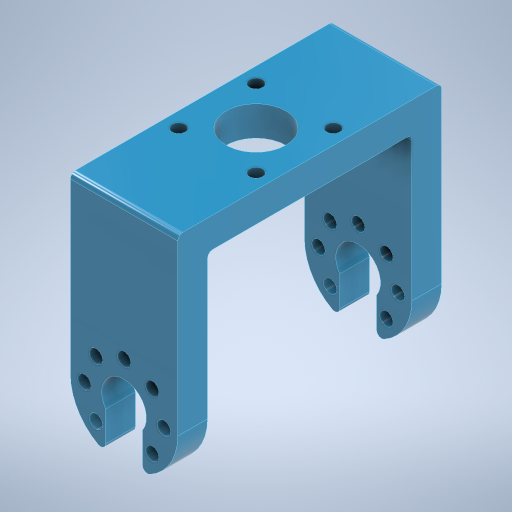
# Autodesk Inventor part: 3D_upper_to_arm1
Saved by Autodesk Inventor 2024 (Build 280153000, 153)
## iProperties
Created: 2024-09-07
Part Number: 3D_upper_to_arm1
Material: PMMA 플라스틱
Document SubType Name: Modeling
Designer: jmha0
Density: 1.188 g/cm^3
Appearance: 하늘색 짙음
Author: jmha0
Autodesk Inventor part; units mm, degrees
ref_plane "YZ Plane" through (0, 0, 0) normal (1, 0, 0) x (0, 1, 0)
ref_plane "XZ Plane" through (0, 0, 0) normal (0, 1, 0) x (-1, 0, 0)
ref_plane "XY Plane" through (0, 0, 0) normal (0, 0, 1) x (1, 0, 0)
sketch "스케치1" plane through (0, 0, 0) normal (0, 0, 1) x (1, 0, 0)
  circle A0 centre (-22.9272, 17.0843) radius 10.8
  circle A1 centre (-22.9272, 17.0843) radius 6
  circle A2 centre (-22.9272, 9.0843) radius 1.05
  circle A3 centre (-28.584, 11.4274) radius 1.05
  circle A4 centre (-30.9272, 17.0843) radius 1.05
  circle A5 centre (-28.584, 22.7411) radius 1.05
  circle A6 centre (-22.9272, 25.0843) radius 1.05
  circle A7 centre (-17.2703, 22.7411) radius 1.05
  circle A8 centre (-14.9272, 17.0843) radius 1.05
  circle A9 centre (-17.2703, 11.4274) radius 1.05
  circle A10 centre (-28.584, 22.7411) radius 1.15
  circle A11 centre (-22.9272, 25.0843) radius 1.15
  circle A12 centre (-17.2703, 22.7411) radius 1.15
  circle A13 centre (-14.9272, 17.0843) radius 1.15
  circle A14 centre (-17.2703, 11.4274) radius 1.15
  circle A15 centre (-28.584, 11.4274) radius 1.15
  circle A16 centre (-30.9272, 17.0843) radius 1.15
  circle A17 centre (-22.9272, 17.0843) radius 3.5
  arc A18 (-19.2272, 17.0843) -> (-26.6272, 17.0843) centre (-22.9272, 17.0843) ccw
  arc A19 (-19.2272, 6.9378) -> (-26.6272, 6.9378) centre (-22.9272, 17.0843) ccw
  line L0 (-26.6272, 17.0843) -> (-26.6272, 6.9378)
  line L1 (-19.2272, 17.0843) -> (-19.2272, 6.9378)
  line L2 (-33.7272, 17.0843) -> (-33.7272, 52.0843)
  line L3 (-12.1272, 17.0843) -> (-12.1272, 52.0843)
  line L4 (-12.1272, 52.0843) -> (-33.7272, 52.0843)
  line L5 (-33.7272, 52.0843) -> (-12.1272, 52.0843)
  line L6 (-12.1272, 52.0843) -> (-12.1272, 58.0843)
  line L7 (-12.1272, 58.0843) -> (-33.7272, 58.0843)
  line L8 (-33.7272, 58.0843) -> (-33.7272, 52.0843)
  point P0 (0, 0)
  dimension "d0" = 0.1
  dimension "d1" = 0.1
  dimension "d2" = 0.1
  dimension "d3" = 0.1
  dimension "d4" = 0.1
  dimension "d5" = 0.1
  dimension "d6" = 0.1
  dimension "d7" = 0.2
  dimension "d8" = 35
  dimension "d9" = 35
  dimension "d10" = 6
  constraints: 20 centre point, 18 end point, 6 point on circle, 6 tangent, 4 parallel, 2 vertical, 1 coincident, 1 concentric, 1 horizontal, 1 perpendicular
  measures "d0" radial gap between concentric circles of A5 A10
  measures "d1" radial gap between concentric circles of A6 A11
  measures "d2" radial gap between concentric circles of A7 A12
  measures "d3" radial gap between concentric circles of A8 A13
  measures "d4" radial gap between concentric circles of A9 A14
  measures "d5" radial gap between concentric circles of A3 A15
  measures "d6" radial gap between concentric circles of A4 A16
  measures "d7" radial gap between concentric circles of A17 A18
  measures "d8" distance of L2.start L4.end
  measures "d9" distance of L3.start L3.end
  measures "d10" distance of L6.end L5.end
extrude "돌출1" add sketch "스케치1" along normal blind 6 contours A0 L1 A1 L0 | A0 L2 L4 L3 | L1 A18 L0 A1 | A3 | A4 | A5 | A6 | A7 | A8 | A9 | A10 | A11 | A12 | A13 | A14 | A15 | A16 picked at (-19.6686, 25.2568) picked at (-26.9638, 14.2707)
sketch "스케치3" plane through (-33.7272, 52.0843, 0) normal (0, 1, 0) x (1, 0, 0)
  line L0 (0, -5.5) -> (21.6, -5.5)
  line L1 (21.6, -5.5) -> (21.6, 0.5)
  line L2 (0, -5.5) -> (0, 0.5)
  line L3 (0, -5.5) -> (21.6, -5.5)
  line L4 (0, -5.5) -> (21.6, -5.5)
  line L5 (21.6, -5.5) -> (21.6, 0.5)
  line L6 (0, -5.5) -> (0, 0.5)
  circle A0 centre (3.0218, -2.5) radius 1.45
  circle A1 centre (18.5782, -2.5) radius 1.45
  line L7 (21.6, 0.5) -> (21.6, 0)
  line L8 (21.6, 0) -> (0, 0)
  line L9 (0, 0) -> (0, 0.5)
  line L10 (21.6, 0) -> (0, 0) projected
  line L11 (0, 0) -> (0, -6) projected
  line L12 (21.6, -6) -> (0, -6) projected
  line L13 (21.6, 0) -> (21.6, -6) projected
  circle A2 centre (10.8, 20.55) radius 6
  line L14 (0, 0) -> (21.6, 0)
  line L15 (21.6, 0) -> (21.6, 41.1)
  line L16 (21.6, 41.1) -> (0, 41.1)
  line L17 (0, 41.1) -> (0, 0)
  line L18 (0, 41.1) -> (21.6, 41.1)
  line L19 (21.6, 41.1) -> (21.6, 47.1)
  line L20 (21.6, 47.1) -> (0, 47.1)
  line L21 (0, 47.1) -> (0, 41.1)
  circle A3 centre (18.5782, 12.7718) radius 1.35
  circle A4 centre (18.5782, 28.3282) radius 1.35
  circle A5 centre (3.0218, 28.3282) radius 1.35
  circle A6 centre (3.0218, 12.7718) radius 1.35
  point P0 (33.7272, 0)
  dimension "d13" = 2.9
  dimension "d14" = 2.9
  dimension "d19" = 0.5
  dimension "d24" = 12
  dimension "d25" = 41.1
  dimension "d26" = 6
  dimension "d29" = 2.7
  dimension "d30" = 2.7
  dimension "d31" = 2.7
  dimension "d32" = 2.7
  constraints: 36 end point, 7 centre point, 5 parallel, 3 horizontal, 2 perpendicular, 1 point on line
  measures "d13" diameter of A0
  measures "d14" diameter of A1
  measures "d19" distance of L7.start L7.end
  measures "d24" diameter of A2
  measures "d25" distance of L15.end L14.end
  measures "d26" distance of L19.end L18.end
  measures "d29" diameter of A3
  measures "d30" diameter of A4
  measures "d31" diameter of A5
  measures "d32" diameter of A6
extrude "돌출2" add sketch "스케치3" against normal blind 6 contours L2 L17 L16 L15 L1 L8
sketch "스케치5" plane through (-12.1272, 52.0843, -41.1) normal (0, 0, -1) x (-1, 0, 0)
  line L0 (19.9594, -6) -> (17.1969, -6) projected
  line L1 (17.1969, 0) -> (19.9594, 0) projected
  line L2 (4.4031, -6) -> (1.6406, -6) projected
  line L3 (1.6406, 0) -> (4.4031, 0) projected
  line L4 (4.4031, -6) -> (1.6406, -6) projected
  line L5 (1.6406, 0) -> (4.4031, 0) projected
  line L6 (0, 0) -> (0, -6) projected
  line L7 (0, 0) -> (21.6, 0) projected
  line L8 (0, 0) -> (0, -6) projected
  line L9 (21.6, -6) -> (0, -6) projected
  line L10 (21.6, 0) -> (21.6, -6) projected
  line L11 (0, 0) -> (21.6, 0) projected
  line L12 (21.6, -6) -> (0, -6) projected
  line L13 (21.6, 0) -> (21.6, -6) projected
  line L14 (19.9594, -6) -> (17.1969, -6) projected
  line L15 (17.1969, 0) -> (19.9594, 0) projected
  arc A0 (14.5, -35) -> (7.1, -35) centre (10.8, -35) ccw projected
  line L16 (16.8, -6) -> (4.8, -6) projected
  line L17 (16.8, -6) -> (4.8, -6) projected
  line L18 (4.8, 0) -> (16.8, 0) projected
  line L19 (4.8, 0) -> (16.8, 0) projected
  line L20 (21.6, -6) -> (0, -6) projected
  line L21 (21.6, -6) -> (0, -6) projected
  line L22 (16.8, -6) -> (4.8, -6) projected
  line L23 (4.8, 0) -> (16.8, 0) projected
  line L24 (0, 0) -> (21.6, 0) projected
  line L25 (0, 0) -> (21.6, 0) projected
  line L26 (21.6, -6) -> (21.6, -35) projected
  line L27 (21.6, 0) -> (21.6, -35) projected
  line L28 (21.6, 0) -> (21.6, -6) projected
  line L29 (0, -35) -> (0, -6) projected
  line L30 (0, 0) -> (0, -6) projected
  line L31 (0, -35) -> (0, 0) projected
  line L32 (1.6406, 0) -> (4.4031, 0) projected
  line L33 (4.4031, -6) -> (1.6406, -6) projected
  line L34 (1.6406, 0) -> (4.4031, 0) projected
  line L35 (17.1969, 0) -> (19.9594, 0) projected
  line L36 (19.9594, -6) -> (17.1969, -6) projected
  line L37 (17.1969, 0) -> (19.9594, 0) projected
  arc A1 (14.5, -35) -> (7.1, -35) centre (10.8, -35) ccw projected
  line L38 (0, -35) -> (0, -6) projected
  line L39 (0, 0) -> (21.6, 0) projected
  line L40 (0, -35) -> (0, 0) projected
  line L41 (19.9594, -6) -> (17.1969, -6) projected
  line L42 (21.6, -6) -> (0, -6) projected
  circle A2 centre (10.8, -12) radius 1.15 projected
  circle A3 centre (5.1431, -14.3431) radius 1.15 projected
  line L43 (21.6, 0) -> (21.6, -35) projected
  circle A4 centre (16.4569, -14.3431) radius 1.15 projected
  circle A5 centre (10.8, -12) radius 1.15 projected
  circle A6 centre (5.1431, -14.3431) radius 1.15 projected
  line L44 (21.6, -6) -> (21.6, -35) projected
  circle A7 centre (16.4569, -14.3431) radius 1.15 projected
  circle A8 centre (5.1431, -25.6569) radius 1.15 projected
  circle A9 centre (5.1431, -25.6569) radius 1.15 projected
  circle A10 centre (5.1431, -25.6569) radius 1.15 projected
  circle A11 centre (5.1431, -25.6569) radius 1.15 projected
  arc A12 (14.5, -45.1464) -> (21.6, -35) centre (10.8, -35) ccw projected
  arc A13 (14.5, -45.1464) -> (21.6, -35) centre (10.8, -35) ccw projected
  line L45 (14.5, -45.1464) -> (14.5, -35) projected
  line L46 (14.5, -45.1464) -> (14.5, -35) projected
  line L47 (7.1, -35) -> (7.1, -45.1464) projected
  line L48 (7.1, -35) -> (7.1, -45.1464) projected
  arc A14 (0, -35) -> (7.1, -45.1464) centre (10.8, -35) ccw projected
  arc A15 (0, -35) -> (7.1, -45.1464) centre (10.8, -35) ccw projected
  circle A16 centre (16.4569, -25.6569) radius 1.15 projected
  circle A17 centre (16.4569, -25.6569) radius 1.15 projected
  circle A18 centre (18.8, -20) radius 1.15 projected
  circle A19 centre (18.8, -20) radius 1.15 projected
  circle A20 centre (10.8, -12) radius 1.15 projected
  circle A21 centre (10.8, -12) radius 1.15 projected
  circle A22 centre (5.1431, -14.3431) radius 1.15 projected
  circle A23 centre (5.1431, -14.3431) radius 1.15 projected
  circle A24 centre (16.4569, -14.3431) radius 1.15 projected
  circle A25 centre (16.4569, -14.3431) radius 1.15 projected
  line L49 (21.6, -6) -> (0, -6) projected
  line L50 (0, -35) -> (0, -6) projected
  arc A26 (0, -35) -> (7.1, -45.1464) centre (10.8, -35) ccw projected
  line L51 (7.1, -35) -> (7.1, -45.1464) projected
  arc A27 (14.5, -35) -> (7.1, -35) centre (10.8, -35) ccw projected
  line L52 (14.5, -45.1464) -> (14.5, -35) projected
  arc A28 (14.5, -45.1464) -> (21.6, -35) centre (10.8, -35) ccw projected
  line L53 (21.6, -6) -> (21.6, -35) projected
  arc A29 (14.5, -45.1464) -> (21.6, -35) centre (10.8, -35) ccw projected
  line L54 (14.5, -45.1464) -> (14.5, -35) projected
  arc A30 (14.5, -35) -> (7.1, -35) centre (10.8, -35) ccw projected
  line L55 (7.1, -35) -> (7.1, -45.1464) projected
  arc A31 (0, -35) -> (7.1, -45.1464) centre (10.8, -35) ccw projected
  line L56 (0, -35) -> (0, 0) projected
  line L57 (0, 0) -> (21.6, 0) projected
  line L58 (21.6, 0) -> (21.6, -35) projected
  arc A32 (14.5, -35) -> (7.1, -35) centre (10.8, -35) ccw projected
  arc A33 (14.5, -35) -> (7.1, -35) centre (10.8, -35) ccw projected
  circle A34 centre (2.8, -20) radius 1.15 projected
  circle A35 centre (2.8, -20) radius 1.15 projected
  circle A36 centre (18.8, -20) radius 1.15 projected
  circle A37 centre (18.8, -20) radius 1.15 projected
  arc A38 (0, -35) -> (7.1, -45.1464) centre (10.8, -35) ccw projected
  arc A39 (0, -35) -> (7.1, -45.1464) centre (10.8, -35) ccw projected
  line L59 (7.1, -35) -> (7.1, -45.1464) projected
  line L60 (7.1, -35) -> (7.1, -45.1464) projected
  arc A40 (14.5, -45.1464) -> (21.6, -35) centre (10.8, -35) ccw projected
  arc A41 (14.5, -45.1464) -> (21.6, -35) centre (10.8, -35) ccw projected
  line L61 (14.5, -45.1464) -> (14.5, -35) projected
  line L62 (14.5, -45.1464) -> (14.5, -35) projected
  circle A42 centre (16.4569, -25.6569) radius 1.15 projected
  circle A43 centre (16.4569, -25.6569) radius 1.15 projected
  line L63 (4.4031, -6) -> (1.6406, -6) projected
  circle A44 centre (2.8, -20) radius 1.05
  circle A45 centre (5.1431, -25.6569) radius 1.05
  circle A46 centre (5.1431, -14.3431) radius 1.05
  circle A47 centre (10.8, -12) radius 1.05
  circle A48 centre (16.4569, -14.3431) radius 1.05
  circle A49 centre (18.8, -20) radius 1.05
  circle A50 centre (16.4569, -25.6569) radius 1.05
  point P0 (-12.1272, -52.0843)
  point P1 (21.6, -6)
  point P2 (0, -6)
  point P3 (21.6, -6)
  point P4 (0, -6)
  point P5 (0, -6)
  dimension "d34" = 0.1
  dimension "d35" = 0.1
  dimension "d36" = 0.1
  dimension "d37" = 0.1
  dimension "d38" = 0.1
  dimension "d39" = 0.1
  constraints: 7 centre point, 8 other
  measures "d34" radial gap between concentric circles of A8 A45
  measures "d35" radial gap between concentric circles of A6 A46
  measures "d36" radial gap between concentric circles of A2 A47
  measures "d37" radial gap between concentric circles of A7 A48
  measures "d38" radial gap between concentric circles of A18 A49
  measures "d39" radial gap between concentric circles of A16 A50
extrude "돌출4" add sketch "스케치5" along normal blind 6 contours L9 L26 A12 L45 A0 L47 A14 L29 L2 L0 | L0 L9 L2 L6 L7 L3 L1 L10 | A2 | A3 | A4 | A8 | A16 | A18 | A34 | A44 | A45 | A46 | A47 | A48 | A49 | A50
sketch "스케치6" plane through (0, 0, 6) normal (0, 0, 1) x (1, 0, 0)
  arc A0 (-33.7272, 17.0843) -> (-26.6272, 6.9378) centre (-22.9272, 17.0843) ccw projected
  line L0 (-26.6272, 6.9378) -> (-26.6272, 17.0843) projected
  arc A1 (-19.2272, 17.0843) -> (-26.6272, 17.0843) centre (-22.9272, 17.0843) ccw projected
  line L1 (-19.2272, 17.0843) -> (-19.2272, 6.9378) projected
  arc A2 (-19.2272, 6.9378) -> (-12.1272, 17.0843) centre (-22.9272, 17.0843) ccw projected
  line L2 (-12.1272, 17.0843) -> (-12.1272, 52.0843) projected
  line L3 (-12.1272, 52.0843) -> (-33.7272, 52.0843) projected
  line L4 (-33.7272, 52.0843) -> (-33.7272, 17.0843) projected
  circle A3 centre (-17.2703, 22.7411) radius 1.05 projected
  circle A4 centre (-22.9272, 25.0843) radius 1.05 projected
  circle A5 centre (-28.584, 22.7411) radius 1.05 projected
  circle A6 centre (-30.9272, 17.0843) radius 1.05 projected
  circle A7 centre (-28.584, 11.4274) radius 1.05 projected
  circle A8 centre (-17.2703, 11.4274) radius 1.05 projected
  circle A9 centre (-14.9272, 17.0843) radius 1.05 projected
  circle A10 centre (-28.584, 22.7411) radius 1.35
  circle A11 centre (-22.9272, 25.0843) radius 1.35
  circle A12 centre (-17.2703, 22.7411) radius 1.35
  circle A13 centre (-14.9272, 17.0843) radius 1.35
  circle A14 centre (-17.2703, 11.4274) radius 1.35
  circle A15 centre (-28.584, 11.4274) radius 1.35
  circle A16 centre (-30.9272, 17.0843) radius 1.35
  point P0 (0, 0)
  dimension "d40" = 2.7
  dimension "d41" = 2.7
  dimension "d42" = 2.7
  dimension "d43" = 2.7
  dimension "d44" = 2.7
  dimension "d45" = 2.7
  dimension "d46" = 2.7
  constraints: 7 centre point, 7 coincident
  measures "d40" diameter of A10
  measures "d41" diameter of A11
  measures "d42" diameter of A12
  measures "d43" diameter of A13
  measures "d44" diameter of A14
  measures "d45" diameter of A15
  measures "d46" diameter of A16
extrude "돌출5" cut sketch "스케치6" against normal blind 100 contours A3 | A4 | A5 | A6 | A7 | A8 | A9 | A10 | A11 | A12 | A13 | A14 | A15 | A16
fillet "모깎기2" radius 1 7 edges at (-26.6272, 6.9378, 3) (-26.6272, 6.9378, -44.1) (-19.2272, 6.9378, 3) (-19.2272, 6.9378, -44.1) (-22.9272, 46.0843, -41.1) (-22.9272, 46.0843, 0) (-22.9272, 52.0843, 6)
sketch "스케치7" plane through (-12.1272, 52.0843, -47.1) normal (0, 0, -1) x (-1, 0, 0)
  circle A0 centre (16.4569, -29.3431) radius 1.35 projected
  circle A1 centre (18.8, -35) radius 1.35 projected
  circle A2 centre (5.1431, -40.6569) radius 1.35 projected
  circle A3 centre (10.8, -27) radius 1.35 projected
  circle A4 centre (5.1431, -29.3431) radius 1.35 projected
  circle A5 centre (16.4569, -40.6569) radius 1.35 projected
  circle A6 centre (2.8, -35) radius 1.35 projected
  line L0 (0, -1) -> (21.6, -1) projected
  line L1 (0, -1) -> (0, -35) projected
  arc A7 (0, -35) -> (5.6204, -44.4769) centre (10.8, -35) ccw projected
  arc A8 (5.6204, -44.4769) -> (7.1, -43.5994) centre (6.1, -43.5994) ccw projected
  line L2 (7.1, -43.5994) -> (7.1, -35) projected
  arc A9 (14.5, -35) -> (7.1, -35) centre (10.8, -35) ccw projected
  line L3 (14.5, -35) -> (14.5, -43.5994) projected
  arc A10 (14.5, -43.5994) -> (15.9796, -44.4769) centre (15.5, -43.5994) ccw projected
  arc A11 (15.9796, -44.4769) -> (21.6, -35) centre (10.8, -35) ccw projected
  line L4 (21.6, -35) -> (21.6, -1) projected
  circle A12 centre (10.8, -35) radius 4.5
  point P0 (-12.1272, -52.0843)
  dimension "d51" = 9
  constraints: 1 centre point, 1 coincident
  measures "d51" diameter of A12
extrude "돌출6" cut sketch "스케치7" against normal blind 100 contours A12 L3 A9 L2 | L2 A9 L3 A12
